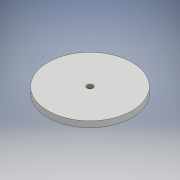
# Autodesk Inventor part: маховик_v1
Saved by Autodesk Inventor 2017.3 (Build 213256000, 256)
## iProperties
Part Number: маховик_v1
Material: Типовые
Document SubType Name: Modeling
Designer: Alexnav
Density: 1 g/cm^3
Appearance: По умолчанию
Mass: 133.808 g
Surface Area: 369.917 cm^2
Volume: 133.808 cm^3
Author: Alexnav
Autodesk Inventor part; units mm, degrees
ref_plane "YZ Plane" through (0, 0, 0) normal (1, 0, 0) x (0, 1, 0)
ref_plane "XZ Plane" through (0, 0, 0) normal (0, 1, 0) x (-1, 0, 0)
ref_plane "XY Plane" through (0, 0, 0) normal (0, 0, 1) x (1, 0, 0)
sketch "Эскиз1" plane through (0, 0, 0) normal (0, 0, 1) x (1, 0, 0)
  circle A0 centre (0, 0) radius 70
  dimension "d0" = 140
  constraints: 1 centre point, 1 coincident
  measures "d0" diameter of A0
extrude "Выдавливание1" add sketch "Эскиз1" along normal blind 10
sketch "Эскиз2" plane through (0, 0, 10) normal (0, 0, 1) x (1, 0, 0)
  circle A0 centre (0, 0) radius 5
  dimension "d3" = 10
  constraints: 1 centre point, 1 coincident
  measures "d3" diameter of A0
extrude "Выдавливание2" cut sketch "Эскиз2" against normal through all
sketch "Эскиз4" plane through (0, 0, 10) normal (0, 0, 1) x (1, 0, 0)
  line L0 (0, -98) -> (0, 98) projected
  circle A0 centre (0, 35) radius 15
  circle A1 centre (-30.3109, 17.5) radius 15
  circle A2 centre (-30.3109, -17.5) radius 15
  circle A3 centre (0, -35) radius 15
  circle A4 centre (30.3109, -17.5) radius 15
  circle A5 centre (30.3109, 17.5) radius 15
  point P0 (0, 0)
  point P1 (0, 0)
  point P2 (0, 0)
  point P3 (0, 0)
  point P4 (0, 0)
  point P5 (0, 0)
  dimension "d9" = 30
  dimension "d10" = 35
  dimension "d13" = 360
  constraints: 6 centre point, 2 coincident, 1 point on line, 17 other
  measures "d9" diameter of A0
  measures "d10" distance of point (0, 0) A0.centre
extrude "Выдавливание3" [suppressed]
